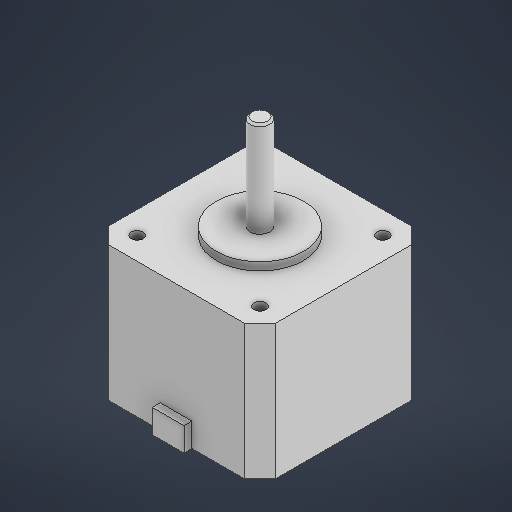
# Autodesk Inventor part: Stepper_motor
Saved by Autodesk Inventor 2026.1 (Build 301233020, 233B)
## iProperties
Created: 2026-03-04
Part Number: Stepper_motor
Material: Generic
Document SubType Name: Modeling
Designer: Mikke
Density: 1 g/cm^3
Appearance: Default
Author: Mikke
Autodesk Inventor part; units mm, degrees
ref_plane "YZ Plane" through (0, 0, 0) normal (1, 0, 0) x (0, 1, 0)
ref_plane "XZ Plane" through (0, 0, 0) normal (0, 1, 0) x (-1, 0, 0)
ref_plane "XY Plane" through (0, 0, 0) normal (0, 0, 1) x (1, 0, 0)
sketch "Sketch1" plane through (0, 0, 0) normal (0, 1, 0) x (-1, 0, 0)
  line L0 (-17.15, 21.15) -> (17.15, 21.15)
  line L1 (21.15, 17.15) -> (21.15, -17.15)
  line L2 (17.15, -21.15) -> (-17.15, -21.15)
  line L3 (-21.15, -17.15) -> (-21.15, 17.15)
  line L4 (-21.15, 21.15) -> (21.15, -21.15) construction
  line L5 (21.15, 21.15) -> (-21.15, -21.15) construction
  line L6 (-15.5, 15.5) -> (15.5, 15.5)
  line L7 (15.5, 15.5) -> (15.5, -15.5)
  line L8 (15.5, -15.5) -> (-15.5, -15.5)
  line L9 (-15.5, -15.5) -> (-15.5, 15.5)
  line L10 (-15.5, 15.5) -> (15.5, -15.5) construction
  line L11 (15.5, 15.5) -> (-15.5, -15.5) construction
  circle A0 centre (15.5, 15.5) radius 1.5
  circle A1 centre (-15.5, 15.5) radius 1.5
  circle A2 centre (15.5, -15.5) radius 1.5
  circle A3 centre (-15.5, -15.5) radius 1.5
  line L12 (21.15, 17.15) -> (17.15, 21.15)
  line L13 (-21.15, 17.15) -> (-17.15, 21.15)
  line L14 (-17.15, -21.15) -> (-21.15, -17.15)
  line L15 (17.15, -21.15) -> (21.15, -17.15)
  point P0 (0, 0)
  dimension "d0" = 42.3
  dimension "d1" = 42.3
  dimension "d2" = 31
  dimension "d3" = 31
  dimension "d4" = 3
  dimension "d7" = 31
  dimension "d10" = 31
  dimension "d13" = 4
  dimension "d14" = 4
  dimension "d15" = 4
  dimension "d16" = 4
  dimension "d17" = 4
  dimension "d18" = 4
  dimension "d19" = 4
  dimension "d20" = 4
  constraints: 32 end point, 8 point on line, 4 centre point, 4 midpoint, 4 parallel, 3 horizontal, 2 perpendicular, 1 coincident, 1 vertical, 6 other
  measures "d0" distance of L4.end L5.end
  measures "d1" distance of L5.start L4.end
  measures "d2" distance of L7.end L8.end
  measures "d3" distance of L6.end L7.end
  measures "d4" diameter of A0
  measures "d7" distance of A0.centre A1.centre
  measures "d10" distance of A0.centre A2.centre
  measures "d13" distance of L1.start L5.start
  measures "d14" distance of L0.end L5.start
  measures "d15" distance of L3.end L4.start
  measures "d16" distance of L0.start L4.start
  measures "d17" distance of L2.end L5.end
  measures "d18" distance of L3.start L5.end
  measures "d19" distance of L2.start L4.end
  measures "d20" distance of L1.end L4.end
extrude "Extrusion1" add sketch "Sketch1" along normal blind 34 contours L0 L12 L1 L15 L2 L14 L3 L13 | L6 A0 L7 A2 L8 A3 L9 A1
sketch "Sketch2" plane through (0, 34, 0) normal (0, 1, 0) x (1, 0, 0)
  circle A0 centre (0, 0) radius 11
  dimension "d23" = 22
  constraints: 1 centre point, 1 coincident
  measures "d23" diameter of A0
extrude "Extrusion2" add sketch "Sketch2" along normal blind 2
sketch "Sketch3" plane through (0, 36, 0) normal (0, 1, 0) x (1, 0, 0)
  circle A0 centre (0, 0) radius 2.5
  dimension "d26" = 5
  constraints: 1 centre point, 1 coincident
  measures "d26" diameter of A0
extrude "Extrusion3" add sketch "Sketch3" along normal blind 24
chamfer "Chamfer1" distance 0.5 angle 45 1 edges at (-2.5, 60, 0)
sketch "Sketch4" plane through (-17.15, 0, 21.15) normal (0, 0, 1) x (1, 0, 0)
  line L0 (13.15, 0) -> (21.15, 0)
  line L1 (0, 0) -> (34.3, 0) projected
  line L2 (21.15, 0) -> (13.15, 0)
  line L3 (13.15, 0) -> (13.15, 6)
  line L4 (13.15, 6) -> (21.15, 6)
  line L5 (21.15, 6) -> (21.15, 0)
  point P0 (17.15, 0)
  dimension "d32" = 8
  dimension "d33" = 8
  dimension "d34" = 6
  constraints: 10 end point, 2 parallel, 1 horizontal, 1 midpoint, 1 perpendicular, 1 point on line
  measures "d32" distance of L0.start L0.end
  measures "d33" distance of L3.end L4.end
  measures "d34" distance of L2.end L3.end
extrude "Extrusion4" add sketch "Sketch4" along normal blind 2
equation "\"d14\" = d13"
equation "\"d15\" = d13"
equation "\"d16\" = d15"
equation "\"d17\" = d13"
equation "\"d18\" = d17"
equation "\"d19\" = d13"
equation "\"d20\" = d19"
body "Solid1"
